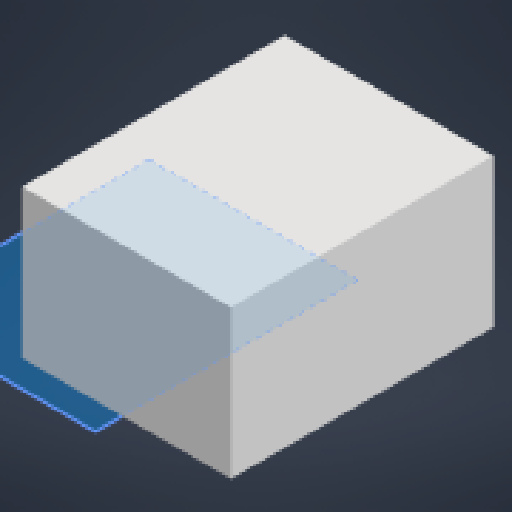
# Autodesk Inventor part: Mold
Saved by Autodesk Inventor 2026 (Build 300175050, 175E)
## iProperties
Created: 2025-08-19
Part Number: Mold
Material: Generic
Document SubType Name: Modeling
Designer: sidsi
Density: 1 g/cm^3
Appearance: Default
Author: sidsi
Autodesk Inventor part; units mm, degrees
ref_plane "YZ Plane" through (0, 0, 0) normal (1, 0, 0) x (0, 1, 0)
ref_plane "XZ Plane" through (0, 0, 0) normal (0, 1, 0) x (-1, 0, 0)
ref_plane "XY Plane" through (0, 0, 0) normal (0, 0, 1) x (1, 0, 0)
ref_plane "Work Plane1" through (1207.234, -74.483, -715.8964) normal (0, 0, -1) x (-1, 0, 0)
sketch "Sketch1" plane through (1207.234, -74.483, -715.8964) normal (0, 0, -1) x (-1, 0, 0)
  line L0 (1061.4617, 729.5034) -> (-81.5383, 729.5034)
  line L1 (-81.5383, 729.5034) -> (-81.5383, -83.2966)
  line L2 (-81.5383, -83.2966) -> (1061.4617, -83.2966)
  line L3 (1061.4617, -83.2966) -> (1061.4617, 729.5034)
  point P0 (1207.234, 74.483)
  dimension "d0" = 1143
  dimension "d1" = 812.8
  constraints: 8 end point, 2 parallel, 1 horizontal, 1 perpendicular
  measures "d0" distance of L0.start L0.end
  measures "d1" distance between parallel lines of L0 L2
extrude "Extrusion1" add sketch "Sketch1" against normal blind 1436.6875
body "Solid1"
